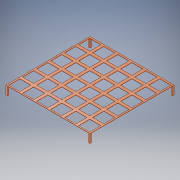
# Autodesk Inventor part: 2ft stand
Saved by Autodesk Inventor 2019 (Build 230136000, 136)
## iProperties
Created: 2020-04-28
Part Number: 2ft stand
Material: Wood (Oak)
Document SubType Name: Modeling
Designer: infinity
Density: 0.76 g/cm^3
Appearance: White Oak - Natural Medium Gloss
Author: infinity
Autodesk Inventor part; units mm, degrees
ref_plane "YZ Plane" through (0, 0, 0) normal (1, 0, 0) x (0, 1, 0)
ref_plane "XZ Plane" through (0, 0, 0) normal (0, 1, 0) x (-1, 0, 0)
ref_plane "XY Plane" through (0, 0, 0) normal (0, 0, 1) x (1, 0, 0)
sketch "Sketch1" plane through (0, 0, 0) normal (0, 1, 0) x (-1, 0, 0)
  line L0 (0, 0) -> (9144, 0)
  line L1 (9144, 0) -> (9144, -9144)
  line L2 (9144, -9144) -> (0, -9144)
  line L3 (0, -9144) -> (0, 0)
  dimension "d0" = 9144
  dimension "d1" = 9144
  constraints: 8 end point, 2 parallel, 1 horizontal, 1 perpendicular
  measures "d0" distance of L0.end L1.end
  measures "d1" distance of L0.start L0.end
extrude "Extrusion1" add sketch "Sketch1" along normal blind 25.4
sketch "Sketch2" plane through (0, 0, 0) normal (0, -1, 0) x (1, 0, 0)
  line L0 (-9144, 0) -> (0, 0) projected
  line L1 (0, 0) -> (-152.4, 0)
  line L2 (-152.4, 0) -> (-152.4, -152.4)
  line L3 (-152.4, -152.4) -> (0, -152.4)
  line L4 (0, -152.4) -> (0, 0)
  line L5 (0, 0) -> (0, -9144) projected
  line L6 (0, -9144) -> (-152.4, -9144)
  line L7 (-152.4, -9144) -> (-152.4, -8991.6)
  line L8 (-152.4, -8991.6) -> (0, -8991.6)
  line L9 (0, -8991.6) -> (0, -9144)
  line L10 (0, -9144) -> (-9144, -9144) projected
  line L11 (-9144, -9144) -> (-8991.6, -9144)
  line L12 (-8991.6, -9144) -> (-8991.6, -8991.6)
  line L13 (-8991.6, -8991.6) -> (-9144, -8991.6)
  line L14 (-9144, -8991.6) -> (-9144, -9144)
  line L15 (-9144, 0) -> (-8991.6, 0)
  line L16 (-8991.6, 0) -> (-8991.6, -152.4)
  line L17 (-8991.6, -152.4) -> (-9144, -152.4)
  line L18 (-9144, -152.4) -> (-9144, 0)
  line L19 (-152.4, -152.4) -> (-8991.6, -152.4) construction
  line L20 (-8991.6, -152.4) -> (-8991.6, -8991.6) construction
  line L21 (-8991.6, -8991.6) -> (-152.4, -8991.6) construction
  line L22 (-152.4, -8991.6) -> (-152.4, -152.4) construction
  line L23 (-9144, 0) -> (-9144, -9144) construction
  point P0 (-4572, -4572)
  dimension "d4" = 152.4
  dimension "d5" = 152.4
  dimension "d6" = 152.4
  dimension "d7" = 152.4
  constraints: 40 end point, 10 parallel, 6 point on line, 5 horizontal, 5 perpendicular
  measures "d4" distance between parallel lines of L0 L19
  measures "d5" distance from line of L0.end L2
  measures "d6" distance between parallel lines of L10 L21
  measures "d7" distance between parallel lines of L23 L20
extrude "Extrusion2" add sketch "Sketch2" along normal blind 914.4
sketch "Sketch3" plane through (0, 25.4, 0) normal (0, 1, 0) x (1, 0, 0)
  line L0 (-8993.1281, 130.2492) -> (-7773.9281, 130.2492)
  line L1 (-7773.9281, 130.2492) -> (-7773.9281, 1349.4492)
  line L2 (-7773.9281, 1349.4492) -> (-8993.1281, 1349.4492)
  line L3 (-8993.1281, 1349.4492) -> (-8993.1281, 130.2492)
  line L4 (-7469.1281, 130.2492) -> (-6249.9281, 130.2492)
  line L5 (-6249.9281, 130.2492) -> (-6249.9281, 1349.4492)
  line L6 (-6249.9281, 1349.4492) -> (-7469.1281, 1349.4492)
  line L7 (-7469.1281, 1349.4492) -> (-7469.1281, 130.2492)
  line L8 (-5945.1281, 130.2492) -> (-4725.9281, 130.2492)
  line L9 (-4725.9281, 130.2492) -> (-4725.9281, 1349.4492)
  line L10 (-4725.9281, 1349.4492) -> (-5945.1281, 1349.4492)
  line L11 (-5945.1281, 1349.4492) -> (-5945.1281, 130.2492)
  line L12 (-4421.1281, 130.2492) -> (-3201.9281, 130.2492)
  line L13 (-3201.9281, 130.2492) -> (-3201.9281, 1349.4492)
  line L14 (-3201.9281, 1349.4492) -> (-4421.1281, 1349.4492)
  line L15 (-4421.1281, 1349.4492) -> (-4421.1281, 130.2492)
  line L16 (-2897.1281, 130.2492) -> (-1677.9281, 130.2492)
  line L17 (-1677.9281, 130.2492) -> (-1677.9281, 1349.4492)
  line L18 (-1677.9281, 1349.4492) -> (-2897.1281, 1349.4492)
  line L19 (-2897.1281, 1349.4492) -> (-2897.1281, 130.2492)
  line L20 (-1373.1281, 130.2492) -> (-153.9281, 130.2492)
  line L21 (-153.9281, 130.2492) -> (-153.9281, 1349.4492)
  line L22 (-153.9281, 1349.4492) -> (-1373.1281, 1349.4492)
  line L23 (-1373.1281, 1349.4492) -> (-1373.1281, 130.2492)
  line L24 (-8993.1281, 1654.2492) -> (-7773.9281, 1654.2492)
  line L25 (-7773.9281, 1654.2492) -> (-7773.9281, 2873.4492)
  line L26 (-7773.9281, 2873.4492) -> (-8993.1281, 2873.4492)
  line L27 (-8993.1281, 2873.4492) -> (-8993.1281, 1654.2492)
  line L28 (-7469.1281, 1654.2492) -> (-6249.9281, 1654.2492)
  line L29 (-6249.9281, 1654.2492) -> (-6249.9281, 2873.4492)
  line L30 (-6249.9281, 2873.4492) -> (-7469.1281, 2873.4492)
  line L31 (-7469.1281, 2873.4492) -> (-7469.1281, 1654.2492)
  line L32 (-5945.1281, 1654.2492) -> (-4725.9281, 1654.2492)
  line L33 (-4725.9281, 1654.2492) -> (-4725.9281, 2873.4492)
  line L34 (-4725.9281, 2873.4492) -> (-5945.1281, 2873.4492)
  line L35 (-5945.1281, 2873.4492) -> (-5945.1281, 1654.2492)
  line L36 (-4421.1281, 1654.2492) -> (-3201.9281, 1654.2492)
  line L37 (-3201.9281, 1654.2492) -> (-3201.9281, 2873.4492)
  line L38 (-3201.9281, 2873.4492) -> (-4421.1281, 2873.4492)
  line L39 (-4421.1281, 2873.4492) -> (-4421.1281, 1654.2492)
  line L40 (-2897.1281, 1654.2492) -> (-1677.9281, 1654.2492)
  line L41 (-1677.9281, 1654.2492) -> (-1677.9281, 2873.4492)
  line L42 (-1677.9281, 2873.4492) -> (-2897.1281, 2873.4492)
  line L43 (-2897.1281, 2873.4492) -> (-2897.1281, 1654.2492)
  line L44 (-1373.1281, 1654.2492) -> (-153.9281, 1654.2492)
  line L45 (-153.9281, 1654.2492) -> (-153.9281, 2873.4492)
  line L46 (-153.9281, 2873.4492) -> (-1373.1281, 2873.4492)
  line L47 (-1373.1281, 2873.4492) -> (-1373.1281, 1654.2492)
  line L48 (-8993.1281, 3178.2492) -> (-7773.9281, 3178.2492)
  line L49 (-7773.9281, 3178.2492) -> (-7773.9281, 4397.4492)
  line L50 (-7773.9281, 4397.4492) -> (-8993.1281, 4397.4492)
  line L51 (-8993.1281, 4397.4492) -> (-8993.1281, 3178.2492)
  line L52 (-7469.1281, 3178.2492) -> (-6249.9281, 3178.2492)
  line L53 (-6249.9281, 3178.2492) -> (-6249.9281, 4397.4492)
  line L54 (-6249.9281, 4397.4492) -> (-7469.1281, 4397.4492)
  line L55 (-7469.1281, 4397.4492) -> (-7469.1281, 3178.2492)
  line L56 (-5945.1281, 3178.2492) -> (-4725.9281, 3178.2492)
  line L57 (-4725.9281, 3178.2492) -> (-4725.9281, 4397.4492)
  line L58 (-4725.9281, 4397.4492) -> (-5945.1281, 4397.4492)
  line L59 (-5945.1281, 4397.4492) -> (-5945.1281, 3178.2492)
  line L60 (-4421.1281, 3178.2492) -> (-3201.9281, 3178.2492)
  line L61 (-3201.9281, 3178.2492) -> (-3201.9281, 4397.4492)
  line L62 (-3201.9281, 4397.4492) -> (-4421.1281, 4397.4492)
  line L63 (-4421.1281, 4397.4492) -> (-4421.1281, 3178.2492)
  line L64 (-2897.1281, 3178.2492) -> (-1677.9281, 3178.2492)
  line L65 (-1677.9281, 3178.2492) -> (-1677.9281, 4397.4492)
  line L66 (-1677.9281, 4397.4492) -> (-2897.1281, 4397.4492)
  line L67 (-2897.1281, 4397.4492) -> (-2897.1281, 3178.2492)
  line L68 (-1373.1281, 3178.2492) -> (-153.9281, 3178.2492)
  line L69 (-153.9281, 3178.2492) -> (-153.9281, 4397.4492)
  line L70 (-153.9281, 4397.4492) -> (-1373.1281, 4397.4492)
  line L71 (-1373.1281, 4397.4492) -> (-1373.1281, 3178.2492)
  line L72 (-8993.1281, 4702.2492) -> (-7773.9281, 4702.2492)
  line L73 (-7773.9281, 4702.2492) -> (-7773.9281, 5921.4492)
  line L74 (-7773.9281, 5921.4492) -> (-8993.1281, 5921.4492)
  line L75 (-8993.1281, 5921.4492) -> (-8993.1281, 4702.2492)
  line L76 (-7469.1281, 4702.2492) -> (-6249.9281, 4702.2492)
  line L77 (-6249.9281, 4702.2492) -> (-6249.9281, 5921.4492)
  line L78 (-6249.9281, 5921.4492) -> (-7469.1281, 5921.4492)
  line L79 (-7469.1281, 5921.4492) -> (-7469.1281, 4702.2492)
  line L80 (-5945.1281, 4702.2492) -> (-4725.9281, 4702.2492)
  line L81 (-4725.9281, 4702.2492) -> (-4725.9281, 5921.4492)
  line L82 (-4725.9281, 5921.4492) -> (-5945.1281, 5921.4492)
  line L83 (-5945.1281, 5921.4492) -> (-5945.1281, 4702.2492)
  line L84 (-4421.1281, 4702.2492) -> (-3201.9281, 4702.2492)
  line L85 (-3201.9281, 4702.2492) -> (-3201.9281, 5921.4492)
  line L86 (-3201.9281, 5921.4492) -> (-4421.1281, 5921.4492)
  line L87 (-4421.1281, 5921.4492) -> (-4421.1281, 4702.2492)
  line L88 (-2897.1281, 4702.2492) -> (-1677.9281, 4702.2492)
  line L89 (-1677.9281, 4702.2492) -> (-1677.9281, 5921.4492)
  line L90 (-1677.9281, 5921.4492) -> (-2897.1281, 5921.4492)
  line L91 (-2897.1281, 5921.4492) -> (-2897.1281, 4702.2492)
  line L92 (-1373.1281, 4702.2492) -> (-153.9281, 4702.2492)
  line L93 (-153.9281, 4702.2492) -> (-153.9281, 5921.4492)
  line L94 (-153.9281, 5921.4492) -> (-1373.1281, 5921.4492)
  line L95 (-1373.1281, 5921.4492) -> (-1373.1281, 4702.2492)
  line L96 (-8993.1281, 6226.2492) -> (-7773.9281, 6226.2492)
  line L97 (-7773.9281, 6226.2492) -> (-7773.9281, 7445.4492)
  line L98 (-7773.9281, 7445.4492) -> (-8993.1281, 7445.4492)
  line L99 (-8993.1281, 7445.4492) -> (-8993.1281, 6226.2492)
  line L100 (-7469.1281, 6226.2492) -> (-6249.9281, 6226.2492)
  line L101 (-6249.9281, 6226.2492) -> (-6249.9281, 7445.4492)
  line L102 (-6249.9281, 7445.4492) -> (-7469.1281, 7445.4492)
  line L103 (-7469.1281, 7445.4492) -> (-7469.1281, 6226.2492)
  line L104 (-5945.1281, 6226.2492) -> (-4725.9281, 6226.2492)
  line L105 (-4725.9281, 6226.2492) -> (-4725.9281, 7445.4492)
  line L106 (-4725.9281, 7445.4492) -> (-5945.1281, 7445.4492)
  line L107 (-5945.1281, 7445.4492) -> (-5945.1281, 6226.2492)
  line L108 (-4421.1281, 6226.2492) -> (-3201.9281, 6226.2492)
  line L109 (-3201.9281, 6226.2492) -> (-3201.9281, 7445.4492)
  line L110 (-3201.9281, 7445.4492) -> (-4421.1281, 7445.4492)
  line L111 (-4421.1281, 7445.4492) -> (-4421.1281, 6226.2492)
  line L112 (-2897.1281, 6226.2492) -> (-1677.9281, 6226.2492)
  line L113 (-1677.9281, 6226.2492) -> (-1677.9281, 7445.4492)
  line L114 (-1677.9281, 7445.4492) -> (-2897.1281, 7445.4492)
  line L115 (-2897.1281, 7445.4492) -> (-2897.1281, 6226.2492)
  line L116 (-1373.1281, 6226.2492) -> (-153.9281, 6226.2492)
  line L117 (-153.9281, 6226.2492) -> (-153.9281, 7445.4492)
  line L118 (-153.9281, 7445.4492) -> (-1373.1281, 7445.4492)
  line L119 (-1373.1281, 7445.4492) -> (-1373.1281, 6226.2492)
  line L120 (-8993.1281, 7750.2492) -> (-7773.9281, 7750.2492)
  line L121 (-7773.9281, 7750.2492) -> (-7773.9281, 8969.4492)
  line L122 (-7773.9281, 8969.4492) -> (-8993.1281, 8969.4492)
  line L123 (-8993.1281, 8969.4492) -> (-8993.1281, 7750.2492)
  line L124 (-7469.1281, 7750.2492) -> (-6249.9281, 7750.2492)
  line L125 (-6249.9281, 7750.2492) -> (-6249.9281, 8969.4492)
  line L126 (-6249.9281, 8969.4492) -> (-7469.1281, 8969.4492)
  line L127 (-7469.1281, 8969.4492) -> (-7469.1281, 7750.2492)
  line L128 (-5945.1281, 7750.2492) -> (-4725.9281, 7750.2492)
  line L129 (-4725.9281, 7750.2492) -> (-4725.9281, 8969.4492)
  line L130 (-4725.9281, 8969.4492) -> (-5945.1281, 8969.4492)
  line L131 (-5945.1281, 8969.4492) -> (-5945.1281, 7750.2492)
  line L132 (-4421.1281, 7750.2492) -> (-3201.9281, 7750.2492)
  line L133 (-3201.9281, 7750.2492) -> (-3201.9281, 8969.4492)
  line L134 (-3201.9281, 8969.4492) -> (-4421.1281, 8969.4492)
  line L135 (-4421.1281, 8969.4492) -> (-4421.1281, 7750.2492)
  line L136 (-2897.1281, 7750.2492) -> (-1677.9281, 7750.2492)
  line L137 (-1677.9281, 7750.2492) -> (-1677.9281, 8969.4492)
  line L138 (-1677.9281, 8969.4492) -> (-2897.1281, 8969.4492)
  line L139 (-2897.1281, 8969.4492) -> (-2897.1281, 7750.2492)
  line L140 (-1373.1281, 7750.2492) -> (-153.9281, 7750.2492)
  line L141 (-153.9281, 7750.2492) -> (-153.9281, 8969.4492)
  line L142 (-153.9281, 8969.4492) -> (-1373.1281, 8969.4492)
  line L143 (-1373.1281, 8969.4492) -> (-1373.1281, 7750.2492)
  point P0 (0, 0)
  dimension "d10" = 1219.2
  dimension "d11" = 1219.2
  dimension "d14" = 1524
  dimension "d17" = 1524
  constraints: 288 end point, 2 collinear, 2 horizontal, 2 parallel, 1 perpendicular, 1 vertical, 278 other
  measures "d10" distance of L2.end L0.start
  measures "d11" distance of L0.start L0.end
  measures "d14" distance of L0.start L4.start
  measures "d17" distance of L0.start L24.start
extrude "Extrusion3" cut sketch "Sketch3" against normal up to surface (25.4 mm away)
equation "\"d1\" = d0"
equation "\"d5\" = d4"
equation "\"d6\" = d4"
equation "\"d7\" = d6"
equation "\"d11\" = d10"
body "Solid1"
